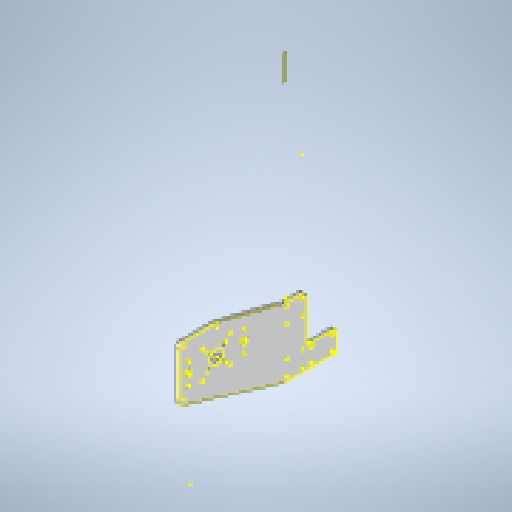
# Autodesk Inventor part: SIDE_SUPPORT_PLATE-PASSIVE
Saved by Autodesk Inventor 2025.2 (Build 292293000, 293)
## iProperties
Created: 2026-02-05
Part Number: SIDE_SUPPORT_PLATE-PASSIVE
Material: Generic
Document SubType Name: Modeling
Designer: composite
Density: 1 g/cm^3
Appearance: Default
Author: composite
Autodesk Inventor part; units mm, degrees
ref_plane "YZ Plane" through (0, 0, 0) normal (1, 0, 0) x (0, 1, 0)
ref_plane "XZ Plane" through (0, 0, 0) normal (0, 1, 0) x (-1, 0, 0)
ref_plane "XY Plane" through (0, 0, 0) normal (0, 0, 1) x (1, 0, 0)
ref_plane "Work Plane1" through (189.9024, 510.8101, -163.2862) normal (-1, 0, 0) x (0, 0, 1)
sketch "Sketch1" plane through (189.9024, 510.8101, -163.2862) normal (-1, 0, 0) x (0, 0, 1)
  arc A0 (-25.9275, -325.719) -> (-33.9275, -333.719) centre (-25.9275, -333.719) ccw projected
  line L0 (-25.9275, -325.719) -> (1.0727, -325.719) projected
  arc A1 (1.0727, -325.719) -> (3.0415, -325.473) centre (1.0727, -317.719) ccw projected
  line L1 (3.0415, -325.473) -> (116.1034, -296.7651) projected
  arc A2 (118.0722, -296.519) -> (116.1034, -296.7651) centre (118.0722, -304.519) ccw projected
  line L2 (118.0722, -296.519) -> (174.0725, -296.519) projected
  arc A3 (182.0725, -304.519) -> (174.0725, -296.519) centre (174.0725, -304.519) ccw projected
  line L3 (182.0725, -304.519) -> (182.0725, -380.5983) projected
  arc A4 (176.4102, -388.2491) -> (182.0725, -380.5983) centre (174.0725, -380.5983) ccw projected
  line L4 (176.4102, -388.2491) -> (3.2153, -441.1698) projected
  arc A5 (0.8775, -441.519) -> (3.2153, -441.1698) centre (0.8775, -433.519) ccw projected
  line L5 (-33.9275, -403.519) -> (-33.9275, -333.719) projected
  circle A6 centre (104.0232, -361.3682) radius 2.25 projected
  circle A7 centre (133.7217, -331.6698) radius 2.25 projected
  circle A8 centre (166.0725, -329.019) radius 2.75 projected
  circle A9 centre (118.8725, -346.519) radius 12 projected
  circle A10 centre (142.4425, -322.949) radius 2.5 projected
  circle A11 centre (-26.9275, -434.819) radius 2.25 projected
  circle A12 centre (-26.9275, -358.419) radius 2.25 projected
  circle A13 centre (-0.9275, -332.419) radius 2.25 projected
  circle A14 centre (-0.9275, -358.419) radius 2.25 projected
  circle A15 centre (71.6725, -346.519) radius 6.05 projected
  circle A16 centre (166.0725, -346.519) radius 6.05 projected
  circle A17 centre (-26.9275, -332.419) radius 2.25 projected
  circle A18 centre (-26.9275, -408.819) radius 2.25 projected
  circle A19 centre (142.4425, -370.089) radius 2.5 projected
  circle A20 centre (95.3025, -370.089) radius 2.5 projected
  circle A21 centre (166.0725, -364.019) radius 2.75 projected
  circle A22 centre (71.6725, -364.019) radius 2.75 projected
  circle A23 centre (133.7217, -361.3682) radius 2.25 projected
  circle A24 centre (104.0232, -331.6698) radius 2.25 projected
  circle A25 centre (71.6725, -329.019) radius 2.75 projected
  circle A26 centre (95.3025, -322.949) radius 2.5 projected
  arc A27 (-81.9275, -405.519) -> (-83.9275, -407.519) centre (-81.9275, -407.519) ccw projected
  line L6 (-81.9275, -405.519) -> (-35.9275, -405.519) projected
  arc A28 (-35.9275, -405.519) -> (-33.9275, -403.519) centre (-35.9275, -403.519) ccw projected
  line L7 (0.8775, -441.519) -> (-81.9275, -441.519) projected
  arc A29 (-83.9275, -439.519) -> (-81.9275, -441.519) centre (-81.9275, -439.519) ccw projected
  line L8 (-83.9275, -439.519) -> (-83.9275, -407.519) projected
  circle A30 centre (-76.4275, -411.519) radius 2.75 projected
  circle A31 centre (-76.4275, -435.519) radius 2.75 projected
  circle A32 centre (-0.9275, -408.819) radius 2.25 projected
  circle A33 centre (-0.9275, -434.819) radius 2.25 projected
  circle A34 centre (-41.4275, -435.519) radius 2.75 projected
  circle A35 centre (-41.4275, -411.519) radius 2.75 projected
  point P0 (163.2862, -510.8101)
  point P1 (-25.9275, -122.4465)
  constraints: 1 other
sketch "Sketch2" plane through (189.9024, 510.8101, -163.2862) normal (-1, 0, 0) x (0, 0, 1)
  line L0 (176.4102, -388.2491) -> (3.2153, -441.1698) projected
  arc A0 (-25.9275, -325.719) -> (-33.9275, -333.719) centre (-25.9275, -333.719) ccw projected
  line L1 (-25.9275, -325.719) -> (1.0727, -325.719) projected
  arc A1 (1.0727, -325.719) -> (3.0415, -325.473) centre (1.0727, -317.719) ccw projected
  line L2 (3.0415, -325.473) -> (116.1034, -296.7651) projected
  circle A2 centre (-0.9275, -332.419) radius 2.25 projected
  circle A3 centre (-0.9275, -358.419) radius 2.25 projected
  circle A4 centre (-26.9275, -332.419) radius 2.25 projected
  circle A5 centre (-26.9275, -358.419) radius 2.25 projected
  arc A6 (0.8775, -441.519) -> (3.2153, -441.1698) centre (0.8775, -433.519) ccw projected
  circle A7 centre (-26.9275, -434.819) radius 2.25 projected
  circle A8 centre (-26.9275, -408.819) radius 2.25 projected
  line L3 (118.0722, -296.519) -> (174.0725, -296.519) projected
  arc A9 (182.0725, -304.519) -> (174.0725, -296.519) centre (174.0725, -304.519) ccw projected
  line L4 (182.0725, -304.519) -> (182.0725, -380.5983) projected
  arc A10 (176.4102, -388.2491) -> (182.0725, -380.5983) centre (174.0725, -380.5983) ccw projected
  arc A11 (118.0722, -296.519) -> (116.1034, -296.7651) centre (118.0722, -304.519) ccw projected
  circle A12 centre (166.0725, -346.519) radius 6.05 projected
  circle A13 centre (166.0725, -364.019) radius 2.75 projected
  circle A14 centre (166.0725, -329.019) radius 2.75 projected
  circle A15 centre (71.6725, -329.019) radius 2.75 projected
  circle A16 centre (71.6725, -364.019) radius 2.75 projected
  circle A17 centre (71.6725, -346.519) radius 6.05 projected
  circle A18 centre (118.8725, -346.519) radius 17.5 construction
  circle A19 centre (131.2468, -334.1446) radius 1.75
  circle A20 centre (106.4981, -334.1446) radius 1.75
  circle A21 centre (106.4981, -358.8934) radius 1.75
  circle A22 centre (131.2468, -358.8934) radius 1.75
  circle A23 centre (118.8725, -346.519) radius 6
  arc A24 (-35.9275, -405.519) -> (-33.9275, -403.519) centre (-35.9275, -403.519) ccw projected
  line L5 (-33.9275, -403.519) -> (-33.9275, -333.719) projected
  circle A25 centre (-41.4275, -411.519) radius 2.75 projected
  circle A26 centre (-41.4275, -435.519) radius 2.75 projected
  line L6 (-81.9275, -405.519) -> (-35.9275, -405.519) projected
  line L7 (0.8775, -441.519) -> (-81.9275, -441.519) projected
  circle A27 centre (-76.4275, -411.519) radius 2.75 projected
  arc A28 (-81.9275, -405.519) -> (-83.9275, -407.519) centre (-81.9275, -407.519) ccw projected
  circle A29 centre (-76.4275, -435.519) radius 2.75 projected
  line L8 (-83.9275, -439.519) -> (-83.9275, -407.519) projected
  arc A30 (-83.9275, -439.519) -> (-81.9275, -441.519) centre (-81.9275, -439.519) ccw projected
  circle A31 centre (-0.9275, -88.6017) radius 2.15 projected
  circle A32 centre (-0.9275, -114.6017) radius 2.15 projected
  circle A33 centre (-0.9275, -408.819) radius 2.25 projected
  circle A34 centre (-0.9275, -434.819) radius 2.25 projected
  point P0 (163.2862, -510.8101)
  point P1 (-25.9275, -122.4465)
  point P2 (163.2862, -510.8101)
  point P3 (-0.9275, -434.819)
  dimension "d2" = 35
  dimension "d3" = 3.5
  dimension "d4" = 90
  dimension "d5" = 12
  constraints: 6 centre point, 4 point on circle, 3 equal radius, 2 coincident, 2 horizontal alignment, 2 vertical alignment
  measures "d2" diameter of A18
  measures "d3" diameter of A19
  measures "d5" diameter of A23
extrude "Extrusion2" add sketch "Sketch2" along normal blind 6 contours L0 A6 L7 A30 L8 A28 L6 A24 L5 A0 L1 A1 L2 A11 L3 A9 L4 A10
body "Solid2"
